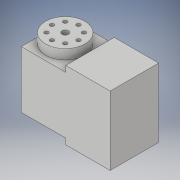
# Autodesk Inventor part: LX-16A
Saved by Autodesk Inventor 2019 (Build 230136000, 136)
## iProperties
Created: 2020-04-05
Part Number: LX-16A
Material: Generic
Document SubType Name: Modeling
Designer: isaac
Density: 1 g/cm^3
Appearance: Default
Author: isaac
Autodesk Inventor part; units mm, degrees
ref_plane "YZ Plane" through (0, 0, 0) normal (1, 0, 0) x (0, 1, 0)
ref_plane "XZ Plane" through (0, 0, 0) normal (0, 1, 0) x (-1, 0, 0)
ref_plane "XY Plane" through (0, 0, 0) normal (0, 0, 1) x (1, 0, 0)
sketch "Sketch1" plane through (0, 0, 0) normal (0, 1, 0) x (-1, 0, 0)
  line L0 (22.6, 12.35) -> (-22.6, 12.35)
  line L1 (-22.6, 12.35) -> (-22.6, -12.35)
  line L2 (-22.6, -12.35) -> (22.6, -12.35)
  line L3 (22.6, -12.35) -> (22.6, 12.35)
  line L4 (22.6, 12.35) -> (-22.6, -12.35) construction
  line L5 (-22.6, 12.35) -> (22.6, -12.35) construction
  point P0 (0, 0)
  dimension "d0" = 45.2
  dimension "d1" = 24.7
  constraints: 12 end point, 2 midpoint, 2 parallel, 1 horizontal, 1 perpendicular
  measures "d0" distance of L2.end L1.end
  measures "d1" distance of L1.end L0.end
extrude "Extrusion1" add sketch "Sketch1" along normal blind 29
sketch "Sketch2" plane through (0, 29, 0) normal (0, 1, 0) x (1, 0, 0)
  line L0 (-22.6, -12.35) -> (22.6, -12.35) construction
  line L1 (-22.6, -12.35) -> (-12.6, -12.35) construction
  line L2 (-12.6, -12.35) -> (-12.6, 0) construction
  line L3 (-12.6, 0) -> (-22.6, 0) construction
  line L4 (-22.6, 0) -> (-22.6, -12.35) construction
  circle A0 centre (-12.6, 0) radius 10
  point P0 (0, 0)
  dimension "d4" = 10
  dimension "d5" = 20
  constraints: 8 end point, 2 parallel, 1 centre point, 1 coincident, 1 horizontal, 1 perpendicular
  measures "d4" distance of L3.end L2.end
  measures "d5" diameter of A0
extrude "Extrusion2" add sketch "Sketch2" along normal blind 5
sketch "Sketch3" plane through (-12.6, 34, 0) normal (0, 1, 0) x (1, 0, 0)
  circle A0 centre (0, 0) radius 6.75 construction
  point P0 (12.6, 0)
  point P1 (-6.75, 0)
  point P2 (-4.773, -4.773)
  point P3 (0, -6.75)
  point P4 (4.773, -4.773)
  point P5 (6.75, 0)
  point P6 (4.773, 4.773)
  point P7 (0, 6.75)
  point P8 (-4.773, 4.773)
  dimension "d8" = 13.5
  dimension "d11" = 360
  constraints: 1 horizontal alignment, 11 other
hole "Hole1" at (-19.35, 34, 0) at (-17.373, 34, 4.773) at (-12.6, 34, 6.75) at (-7.827, 34, 4.773) at (-5.85, 34, 0) at (-7.827, 34, -4.773) at (-12.6, 34, -6.75) at (-17.373, 34, -4.773) direction (0, -1, 0) diameter 2 depth 5 tip angle 118
sketch "Sketch4" plane through (-12.6, 34, 0) normal (0, 1, 0) x (1, 0, 0)
  point P0 (12.6, 0)
  point P1 (0, 0)
hole "Hole2" at (-12.6, 34, 0) direction (0, -1, 0) diameter 3.25 depth 5 tip angle 118
sketch "Sketch5" plane through (0, 0, 0) normal (0, -1, 0) x (1, 0, 0)
  line L0 (22.6, -12.35) -> (-22.6, -12.35) construction
  line L1 (-22.6, -12.35) -> (-12.6, -12.35) construction
  line L2 (-12.6, -12.35) -> (-12.6, 0) construction
  line L3 (-12.6, 0) -> (-22.6, 0) construction
  line L4 (-22.6, 0) -> (-22.6, -12.35) construction
  circle A0 centre (-12.6, 0) radius 10 construction
  circle A1 centre (-12.6, 0) radius 3
  point P0 (0, 0)
  dimension "d27" = 10
  dimension "d28" = 6
  constraints: 8 end point, 2 parallel, 1 centre point, 1 coincident, 1 horizontal, 1 horizontal alignment, 1 perpendicular
  measures "d27" distance of L3.end L2.end
  measures "d28" diameter of A1
extrude "Extrusion3" add sketch "Sketch5" along normal blind 4
sketch "Sketch6" plane through (-12.6, -4, 0) normal (0, -1, 0) x (1, 0, 0)
  point P0 (12.6, 0)
  point P1 (0, 0)
hole "Hole3" at (-12.6, -4, 0) direction (0, 1, 0) diameter 2.75 depth 4 tip angle 118
sketch "Sketch7" plane through (0, 29, 0) normal (0, 1, 0) x (1, 0, 0)
  line L0 (-22.6, -12.35) -> (22.6, -12.35) projected
  line L1 (22.6, -12.35) -> (22.6, 12.35) projected
  line L2 (0, -12.35) -> (22.6, -12.35)
  line L3 (22.6, -12.35) -> (22.6, 12.35)
  line L4 (22.6, 12.35) -> (0, 12.35)
  line L5 (0, 12.35) -> (0, -12.35)
  point P0 (0, 0)
  constraints: 8 end point, 2 parallel, 1 horizontal, 1 midpoint, 1 perpendicular
extrude "Extrusion4" add sketch "Sketch7" along normal blind 3
sketch "Sketch8" plane through (0, 0, 0) normal (0, -1, 0) x (1, 0, 0)
  line L0 (22.6, -12.35) -> (-22.6, -12.35) projected
  line L1 (22.6, 12.35) -> (22.6, -12.35) projected
  line L2 (0, -12.35) -> (22.6, -12.35)
  line L3 (22.6, -12.35) -> (22.6, 12.35)
  line L4 (22.6, 12.35) -> (0, 12.35)
  line L5 (0, 12.35) -> (0, -12.35)
  point P0 (0, 0)
  constraints: 8 end point, 2 parallel, 1 horizontal, 1 midpoint, 1 perpendicular
extrude "Extrusion5" add sketch "Sketch8" along normal blind 3
body "Solid1"
